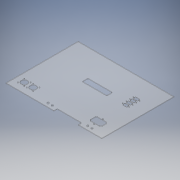
# Autodesk Inventor part: Top_Acrylic_Mount
Saved by Autodesk Inventor 2019 (Build 230136000, 136)
## iProperties
Created: 2019-05-23
Part Number: Top_Acrylic_Mount
Material: PET Plastic
Document SubType Name: Modeling
Designer: Jorian Bruslind
Density: 1.541 g/cm^3
Appearance: Polycarbonate - Clear
Author: Jorian Bruslind
Autodesk Inventor part; units mm, degrees
ref_plane "YZ Plane" through (0, 0, 0) normal (1, 0, 0) x (0, 1, 0)
ref_plane "XZ Plane" through (0, 0, 0) normal (0, 1, 0) x (-1, 0, 0)
ref_plane "XY Plane" through (0, 0, 0) normal (0, 0, 1) x (1, 0, 0)
sketch "Sketch1" plane through (0, 0, 0) normal (0, 1, 0) x (-1, 0, 0)
  line L0 (0, 0) -> (433, 0)
  line L1 (433, 0) -> (433, -326)
  line L2 (433, -326) -> (0, -326)
  line L3 (0, -326) -> (0, 0)
  dimension "d0" = 433
  dimension "d1" = 326
  constraints: 8 end point, 2 parallel, 1 horizontal, 1 perpendicular
  measures "d0" distance of L1.end L2.end
  measures "d1" distance of L0.end L1.end
extrude "Extrusion1" add sketch "Sketch1" along normal blind 3
sketch "Sketch2" plane through (0, 3, 0) normal (0, 1, 0) x (1, 0, 0)
  line L0 (0, 0) -> (0, 326) projected
  line L1 (0, 326) -> (-10, 326)
  line L2 (0, 326) -> (-433, 326) projected
  line L3 (-10, 326) -> (-10, 316)
  circle A0 centre (-10, 316) radius 1.75
  circle A1 centre (-423, 316) radius 1.75
  circle A2 centre (-10, 11) radius 1.75
  circle A3 centre (-423, 11) radius 1.75
  dimension "d4" = 10
  dimension "d5" = 10
  dimension "d6" = 3.5
  dimension "d9" = 413
  dimension "d12" = 305
  constraints: 4 centre point, 4 end point, 1 coincident, 1 horizontal, 1 perpendicular, 1 point on line, 1 vertical, 6 other
  measures "d4" distance of L0.end L1.end
  measures "d5" distance of L1.end L3.end
  measures "d6" diameter of A0
  measures "d9" distance of A0.centre A1.centre
  measures "d12" distance of A0.centre A2.centre
extrude "Extrusion2" [suppressed]
sketch "Sketch3" plane through (0, 3, 0) normal (0, 1, 0) x (1, 0, 0)
  line L0 (-433, 0) -> (0, 0) projected
  line L1 (0, 0) -> (-156, 0)
  line L2 (-156, 0) -> (-156, 178.5)
  line L3 (-156, 178.5) -> (-266.2, 178.5)
  line L4 (-266.2, 178.5) -> (-266.2, 203.5)
  line L5 (-266.2, 203.5) -> (-156, 203.5)
  line L6 (-156, 203.5) -> (-156, 178.5)
  dimension "d17" = 156
  dimension "d18" = 178.5
  dimension "d19" = 90
  dimension "d20" = 110.2
  dimension "d21" = 25
  constraints: 12 end point, 2 parallel, 2 perpendicular, 1 horizontal, 1 point on line
  measures "d17" distance of L0.end L1.end
  measures "d18" distance of L1.end L2.end
  measures "d19" angle of L1 L2
  measures "d20" distance of L4.end L5.end
  measures "d21" distance of L3.end L4.end
extrude "Extrusion3" cut sketch "Sketch3" against normal blind 3
sketch "Sketch4" plane through (0, 3, 0) normal (0, 1, 0) x (1, 0, 0)
  line L0 (0, 0) -> (-106, 0)
  line L1 (-156, 178.5) -> (-156, 203.5) projected
  line L2 (-106, 0) -> (-216.2, 0)
  line L3 (-216.2, 0) -> (-216.2, 15)
  line L4 (-216.2, 15) -> (-106, 15)
  line L5 (-106, 15) -> (-106, 0)
  dimension "d24" = 110.2
  dimension "d25" = 15
  constraints: 10 end point, 2 parallel, 2 perpendicular, 1 horizontal
  measures "d24" distance of L3.end L4.end
  measures "d25" distance of L2.end L3.end
extrude "Extrusion5" cut sketch "Sketch4" against normal blind 3
sketch "Sketch5" plane through (0, 3, 0) normal (0, 1, 0) x (1, 0, 0)
  line L0 (-106, 0) -> (0, 0) projected
  line L1 (0, 0) -> (0, 326) projected
  arc A0 (-241.2, 10) -> (-241.2, 25) centre (-241.2, 17.5) ccw
  line L2 (-433, 0) -> (-216.2, 0) projected
  line L3 (-216.2, 0) -> (-216.2, 15) projected
  line L4 (-241.2, 10) -> (-260.2, 10)
  line L5 (-241.2, 25) -> (-260.2, 25)
  arc A1 (-260.2, 25) -> (-260.2, 10) centre (-260.2, 17.5) ccw
  line L6 (-106, 15) -> (-216.2, 15) projected
  line L7 (-161.1, 15) -> (-161.1, 25)
  line L8 (-260.2, 27) -> (-241.2, 27)
  arc A2 (-241.2, 8) -> (-241.2, 27) centre (-241.2, 17.5) ccw
  line L9 (-241.2, 8) -> (-260.2, 8)
  arc A3 (-260.2, 27) -> (-260.2, 8) centre (-260.2, 17.5) ccw
  line L10 (-62, 27) -> (-81, 27)
  arc A4 (-81, 27) -> (-81, 8) centre (-81, 17.5) ccw
  line L11 (-81, 8) -> (-62, 8)
  arc A5 (-62, 8) -> (-62, 27) centre (-62, 17.5) ccw
  circle A6 centre (-409.063, 30) radius 2
  line L12 (-433, 326) -> (-433, 0) projected
  line L13 (-433, 25) -> (-433, 26)
  circle A7 centre (-380.488, 30) radius 2
  circle A8 centre (-409.063, 58.575) radius 2
  circle A9 centre (-380.488, 58.575) radius 2
  line L14 (-380.488, 30) -> (-374.7755, 30)
  line L15 (-374.7755, 30) -> (-374.7755, 26)
  circle A10 centre (-340.488, 30) radius 2
  circle A11 centre (-369.063, 30) radius 2
  circle A12 centre (-340.488, 58.575) radius 2
  circle A13 centre (-369.063, 58.575) radius 2
  circle A14 centre (-260.2, 17.5) radius 4
  circle A15 centre (-241.2, 17.5) radius 4
  circle A16 centre (-81, 17.5) radius 4
  circle A17 centre (-62, 17.5) radius 4
  dimension "d48" = 25
  dimension "d49" = 7.5
  dimension "d50" = 15
  dimension "d51" = 19
  dimension "d52" = 19
  dimension "d53" = 10
  dimension "d54" = 7.5
  dimension "d55" = 10
  dimension "d57" = 2
  dimension "d58" = 4
  dimension "d59" = 1
  dimension "d62" = 28.575
  dimension "d65" = 28.575
  dimension "d68" = 30
  dimension "d69" = 23.937
  dimension "d70" = 5.7125
  dimension "d71" = 4
  dimension "d74" = 8
  dimension "d75" = 8
  dimension "d76" = 8
  dimension "d77" = 8
  constraints: 20 end point, 18 centre point, 12 point on circle, 10 symmetric about line, 4 coincident, 4 horizontal, 2 point on line, 2 vertical, 1 midpoint, 1 perpendicular, 15 other
  measures "d48" distance from line of L3 A0.centre
  measures "d49" radius of A0
  measures "d50" distance of L4.start L5.start
  measures "d51" distance of L4.start L4.end
  measures "d52" distance of L5.start L5.end
  measures "d53" distance between parallel lines of L4 L2
  measures "d54" radius of A1
  measures "d55" distance of L7.start L7.end
  measures "d57" distance between parallel lines of L5 L8
  measures "d58" diameter of A6
  measures "d59" distance of L13.start L13.end
  measures "d62" distance of A6.centre L14.start
  measures "d65" distance of A6.centre A8.centre
  measures "d68" distance from line of L2 A6.centre
  measures "d69" distance from line of L12 A6.centre
  measures "d70" distance of L14.start L14.end
  measures "d71" distance of L14.end L15.end
  measures "d74" diameter of A14
  measures "d75" diameter of A15
  measures "d76" diameter of A16
  measures "d77" diameter of A17
sketch "Sketch6" plane through (0, 3, 0) normal (0, 1, 0) x (1, 0, 0)
  line L0 (-368.00851, 48.3515) -> (-368.00851, 40.2235)
  arc A0 (-368.00851, 40.2235) -> (-360.567591, 31.7145) centre (-354.7755, 44.2875) ccw
  line L1 (-360.567591, 31.7145) -> (-348.983409, 31.7145)
  arc A1 (-348.983409, 31.7145) -> (-368.00851, 48.3515) centre (-354.7755, 44.2875) ccw
  point P0 (0, 0)
extrude "Extrusion8" cut sketch "Sketch6" against normal blind 10
sketch "Sketch7" plane through (0, 3, 0) normal (0, 1, 0) x (1, 0, 0)
  line L0 (-400.567591, 31.7145) -> (-388.983409, 31.7145)
  arc A0 (-408.00851, 40.2235) -> (-400.567591, 31.7145) centre (-394.7755, 44.2875) ccw
  line L1 (-408.00851, 48.3515) -> (-408.00851, 40.2235)
  arc A1 (-388.983409, 31.7145) -> (-408.00851, 48.3515) centre (-394.7755, 44.2875) ccw
  spline S0 degree 3 poles (-389.406938, 54.823898) (-388.390749, 54.267547) (-387.460994, 53.564387) (-385.84343, 51.912919) (-385.165613, 50.978524) (-383.943022, 48.630058) (-383.513602, 47.173446) (-383.242245, 44.199297) (-383.395869, 42.708972) (-384.162923, 40.212592) (-384.65198, 39.192577) (-385.90968, 37.341595) (-386.670794, 36.51622) (-387.542022, 35.818205) knots -2.26150463 -2.26150463 -2.26150463 -2.26150463 -1.91444355 -1.91444355 -1.56975978 -1.56975978 -1.11906729 -1.11906729 -0.67340462 -0.67340462 -0.33491211 -0.33491211 -0.00000362 -0.00000362 -0.00000362 -0.00000362
  spline S1 degree 3 poles (-405.311241, 49.657311) (-404.984037, 50.299123) (-404.59925, 50.909354) (-404.161857, 51.480149) (-403.592618, 52.223003) (-402.935001, 52.897725) (-402.207177, 53.485765) (-401.479343, 54.073813) (-400.681277, 54.575116) (-399.835668, 54.975465) (-398.990055, 55.375817) (-398.09639, 55.675429) (-397.180343, 55.865696) (-396.264298, 56.055963) (-395.325283, 56.137018) (-394.390134, 56.106527) (-393.454987, 56.076036) (-392.523302, 55.934) (-391.62154, 55.684448) (-390.857007, 55.472874) (-390.114492, 55.184331) (-389.406936, 54.823903) knots 0.00007576 0.00007576 0.00007576 0.00007576 0.11620202 0.11620202 0.11620202 0.26733283 0.26733283 0.26733283 0.41846585 0.41846585 0.41846585 0.56959968 0.56959968 0.56959968 0.72073311 0.72073311 0.72073311 0.87186623 0.87186623 0.87186623 0.99999994 0.99999994 0.99999994 0.99999994
  spline S2 degree 3 poles (-405.311241, 49.657311) (-405.311453, 49.656894) (-405.311665, 49.656478) (-405.311865, 49.656056) knots 0 0 0 0 1 1 1 1
  spline S3 degree 3 poles (-398.242768, 33.616347) (-399.101657, 33.866229) (-399.928425, 34.217566) (-401.4887, 35.114232) (-402.215923, 35.656592) (-403.881846, 37.239986) (-404.783721, 38.451542) (-406.090297, 41.375417) (-406.393813, 42.874449) (-406.463274, 45.210582) (-406.381068, 46.132061) (-406.003821, 47.938759) (-405.706493, 48.820994) (-405.311865, 49.656056) knots -1.93513042 -1.93513042 -1.93513042 -1.93513042 -1.66485342 -1.66485342 -1.39364751 -1.39364751 -0.97417983 -0.97417983 -0.55134806 -0.55134806 -0.27708825 -0.27708825 -0.00000481 -0.00000481 -0.00000481 -0.00000481
  line L2 (-398.242768, 33.616347) -> (-398.2173, 33.694728)
  arc A2 (-398.2173, 33.694728) -> (-387.542003, 35.818182) centre (-394.7755, 44.2875) ccw
  point P0 (0, 0)
extrude "Extrusion9" cut sketch "Sketch7" against normal blind 10 contours A0 L1 A1 L0 | S0 A2 L2 S3 S1
fillet "Fillet1" radius 2 4 edges at (-266.2, 1.5, -203.5) (-156, 1.5, -203.5) (-156, 1.5, -178.5) (-266.2, 1.5, -178.5)
extrude "Extrusion10" cut sketch "Sketch5" against normal blind 10 contours A6 | A7 | A8 | A9 | A10 | A11 | A12 | A13 | A14 | A15 | A16 | A17
sketch "Sketch8" plane through (0, 3, 0) normal (0, 1, 0) x (1, 0, 0)
  line L0 (-56, 45) -> (-94.9, 45)
  line L1 (-50, 51) -> (-56, 45)
  line L2 (-50, 66) -> (-50, 51)
  line L3 (-56, 72) -> (-50, 66)
  line L4 (-64.5, 72) -> (-57.5, 72)
  line L5 (-94.9, 72) -> (-64.5, 72)
  line L6 (-64.5, 72) -> (-57.5, 72)
  line L7 (-57.5, 72) -> (-56, 72)
  line L8 (-95.7, 70.62) -> (-95.7, 46.38)
  line L9 (-96.9, 47) -> (-96.9, 70)
  line L10 (-95.7, 70.62) -> (-95.7, 46.38)
  arc A0 (-96.9, 47) -> (-94.9, 45) centre (-94.9, 47) ccw
  arc A1 (-94.9, 72) -> (-96.9, 70) centre (-94.9, 70) ccw
  line L11 (-64.5, 74) -> (-94.9, 74)
  arc A2 (-94.9, 74) -> (-98.9, 70) centre (-94.9, 70) ccw
  line L12 (-98.9, 70) -> (-98.9, 47)
  arc A3 (-98.9, 47) -> (-94.9, 43) centre (-94.9, 47) ccw
  line L13 (-94.9, 43) -> (-55.171573, 43)
  line L14 (-55.171573, 43) -> (-48, 50.171573)
  line L15 (-48, 50.171573) -> (-48, 66.828427)
  line L16 (-48, 66.828427) -> (-55.171573, 74)
  line L17 (-55.171573, 74) -> (-57.5, 74)
  line L18 (-64.5, 74) -> (-57.5, 74)
  circle A4 centre (-73.45, 38.5) radius 2.25
  circle A5 centre (-73.45, 78.5) radius 2.25
  point P0 (0, 0)
  dimension "d87" = 2
  constraints: 16 end point, 4 point on circle, 2 centre point, 1 horizontal, 8 other
  measures "d87" distance between parallel lines of L5 L11
extrude "Extrusion11" cut sketch "Sketch8" against normal blind 3 contours L0 A0 L9 A1 L5 L4 L7 L3 L2 L1 | L18 L17 L16 L15 L14 L13 A3 L12 A2 L11 | A4 | A5
sketch "Sketch9" plane through (0, 3, 0) normal (0, 1, 0) x (1, 0, 0)
  line L0 (-85.15475, 179.9085) -> (-85.15475, 189.5605)
  line L1 (-65.20305, 179.7434) -> (-87.19945, 179.7434)
  line L2 (-66.2, 178.9814) -> (-66.2, 190.4876)
  line L3 (-87.19945, 189.7256) -> (-65.20305, 189.7256)
  line L4 (-86.2025, 178.9814) -> (-86.2025, 190.4876)
  line L5 (-67.24775, 189.5605) -> (-67.24775, 179.9085)
  line L6 (-86.2025, 195.4876) -> (-86.2025, 206.9938)
  line L7 (-66.2, 206.9938) -> (-86.2025, 206.9938)
  line L8 (-66.2, 195.4876) -> (-66.2, 206.9938)
  line L9 (-66.2, 195.4876) -> (-86.2025, 195.4876)
  line L10 (-66.2, 211.9938) -> (-86.2025, 211.9938)
  line L11 (-86.2025, 211.9938) -> (-86.2025, 223.5)
  line L12 (-66.2, 223.5) -> (-86.2025, 223.5)
  line L13 (-66.2, 211.9938) -> (-66.2, 223.5)
  circle A0 centre (-73.45, 78.5) radius 2.25
  circle A1 centre (-73.45, 38.5) radius 2.25
  arc A2 (-94.9, 74) -> (-98.9, 70) centre (-94.9, 70) ccw
  line L14 (-94.9, 74) -> (-55.171573, 74)
  line L15 (-55.171573, 74) -> (-48, 66.828427)
  line L16 (-48, 66.828427) -> (-48, 50.171573)
  line L17 (-48, 50.171573) -> (-55.171573, 43)
  line L18 (-55.171573, 43) -> (-94.9, 43)
  arc A3 (-98.9, 47) -> (-94.9, 43) centre (-94.9, 47) ccw
  line L19 (-98.9, 47) -> (-98.9, 70)
  circle A4 centre (-81, 17.5) radius 4
  circle A5 centre (-260.2, 17.5) radius 4
  circle A6 centre (-340.488, 58.575) radius 2
  circle A7 centre (-369.063, 30) radius 2
  circle A8 centre (-409.063, 58.575) radius 2
  circle A9 centre (-409.063, 30) radius 2
  circle A10 centre (-380.488, 30) radius 2
  circle A11 centre (-380.488, 58.575) radius 2
  circle A12 centre (-340.488, 30) radius 2
  circle A13 centre (-369.063, 58.575) radius 2
  circle A14 centre (-241.2, 17.5) radius 4
  circle A15 centre (-62, 17.5) radius 4
  arc A16 (-388.983409, 31.7145) -> (-408.00851, 48.3515) centre (-394.7755, 44.2875) ccw
  line L20 (-388.983409, 31.7145) -> (-400.567591, 31.7145)
  arc A17 (-408.00851, 40.2235) -> (-400.567591, 31.7145) centre (-394.7755, 44.2875) ccw
  line L21 (-408.00851, 40.2235) -> (-408.00851, 48.3515)
  arc A18 (-368.00851, 40.2235) -> (-360.567591, 31.7145) centre (-354.7755, 44.2875) ccw
  line L22 (-368.00851, 40.2235) -> (-368.00851, 48.3515)
  arc A19 (-348.983409, 31.7145) -> (-368.00851, 48.3515) centre (-354.7755, 44.2875) ccw
  line L23 (-348.983409, 31.7145) -> (-360.567591, 31.7145)
  line L24 (-106, 15) -> (-106, 0)
  line L25 (-106, 0) -> (0, 0)
  line L26 (0, 0) -> (0, 326)
  line L27 (0, 326) -> (-433, 326)
  line L28 (-433, 326) -> (-433, 0)
  line L29 (-433, 0) -> (-216.2, 0)
  line L30 (-216.2, 0) -> (-216.2, 15)
  line L31 (-216.2, 15) -> (-106, 15)
  line L32 (-264.2, 203.5) -> (-158, 203.5)
  arc A20 (-156, 201.5) -> (-158, 203.5) centre (-158, 201.5) ccw
  line L33 (-156, 201.5) -> (-156, 180.5)
  arc A21 (-158, 178.5) -> (-156, 180.5) centre (-158, 180.5) ccw
  line L34 (-158, 178.5) -> (-264.2, 178.5)
  arc A22 (-266.2, 180.5) -> (-264.2, 178.5) centre (-264.2, 180.5) ccw
  line L35 (-266.2, 180.5) -> (-266.2, 201.5)
  arc A23 (-264.2, 203.5) -> (-266.2, 201.5) centre (-264.2, 201.5) ccw
  circle A24 centre (-90.78135, 217.7469) radius 1.4478
  circle A25 centre (-90.78135, 201.2407) radius 1.4478
  circle A26 centre (-90.78135, 184.7345) radius 1.4478
  circle A27 centre (-61.62115, 184.7345) radius 1.4478
  circle A28 centre (-61.62115, 201.2407) radius 1.4478
  circle A29 centre (-61.62115, 217.7469) radius 1.4478
  line L36 (-86.2025, 238.5) -> (-66.2, 238.5)
  line L37 (-86.2025, 226.9938) -> (-66.2, 226.9938)
  line L38 (-86.2025, 238.5) -> (-86.2025, 226.9938)
  line L39 (-66.2, 238.5) -> (-66.2, 226.9938)
  circle A30 centre (-61.62115, 232.7469) radius 1.4478
  circle A31 centre (-90.78135, 232.7469) radius 1.4478
  line L40 (-66.2, 178.9814) -> (-86.2025, 178.9814)
  line L41 (-66.2, 190.4876) -> (-86.2025, 190.4876)
extrude "Extrusion12" cut sketch "Sketch9" against normal blind 3 contours L2 L40 L4 L1 | L1 L4 L3 L2 | L3 L4 L41 L2 | L6 L7 L8 L9 | L10 L11 L12 L13 | A24 | A25 | A26 | A27 | A28 | A29 | L36 L39 L37 L38 | A30 | A31
fillet "Fillet2" radius 4 18 edges at (-216.2, 1.5, -15) (-106, 1.5, -15) (-66.2, 1.5, -238.5) (-66.2, 1.5, -226.9938) (-86.2025, 1.5, -238.5) (-86.2025, 1.5, -226.9938) (-86.2025, 1.5, -211.9938) (-86.2025, 1.5, -223.5) (-66.2, 1.5, -223.5) (-66.2, 1.5, -211.9938) (-66.2, 1.5, -195.4876) (-66.2, 1.5, -206.9938) (-86.2025, 1.5, -206.9938) (-86.2025, 1.5, -195.4876) (-86.2025, 1.5, -178.9814) (-86.2025, 1.5, -190.4876) (-66.2, 1.5, -178.9814) (-66.2, 1.5, -190.4876)
body "Solid1"
